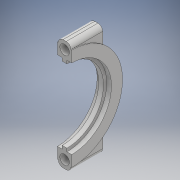
# Autodesk Inventor part: Upper lower eccentric trap (2)
Saved by Autodesk Inventor 2017 (Build 210142000, 142)
## iProperties
Created: 2018-11-20
Part Number: Upper lower eccentric trap (2)
Material: Generic
Document SubType Name: Modeling
Designer: Arman Grewal
Density: 1 g/cm^3
Appearance: Default
Author: Arman Grewal
Autodesk Inventor part; units mm, degrees
ref_plane "XZ Plane" through (0, 0, 0) normal (0, 1, 0) x (-1, 0, 0)
ref_plane "XY Plane" through (0, 0, 0) normal (0, 0, 1) x (1, 0, 0)
sketch "Sketch1" plane through (0, 0, 0) normal (1, 0, 0) x (0, 1, 0)
  arc A0 (0, -16) -> (0, 16) centre (0, 0) ccw construction
  arc A1 (0, -16) -> (0, 16) centre (0, 0) ccw
  arc A2 (0, -12.5) -> (0, 12.5) centre (0, 0) ccw
  line L0 (0, 12.5) -> (0, 16)
  line L1 (0, -12.5) -> (0, -16)
  dimension "d0" = 32
  dimension "d1" = 25
  dimension "d2" = 0
  dimension "d3" = 0
  dimension "d4" = 0
  dimension "d5" = 16
  constraints: 6 point on circle, 4 end point, 3 centre point, 3 coincident, 1 collinear, 1 concentric, 1 vertical
  measures "d0" diameter of A0
  measures "d1" diameter of A2
  measures "d2" distance between parallel lines of L0 L1
  measures "d3" distance from line of point (0, 0) L0
  measures "d4" distance from line of point (0, 0) L0
  measures "d5" distance of point (0, 0) L0.end
extrude "Extrusion1" add sketch "Sketch1" along normal blind 4.5
ref_plane "Work Plane1" through (2.25, 0, 0) normal (1, 0, 0) x (0, 1, 0)
sketch "Sketch3" plane through (2.25, 0, 0) normal (1, 0, 0) x (0, 1, 0)
  arc A0 (0, -12.5) -> (0, 12.5) centre (0, 0) ccw projected
  arc A1 (0, -11.5) -> (0, 11.5) centre (0, 0) ccw
  line L0 (0, -11.5) -> (0, -12.5)
  line L1 (0, 12.5) -> (0, 11.5)
  dimension "d8" = 23
  constraints: 4 end point, 2 point on circle, 2 vertical, 1 centre point, 1 concentric
  measures "d8" diameter of A1
extrude "Extrusion2" add sketch "Sketch3" along normal mid plane 1.5
sketch "Sketch4" plane through (0, 0, 12.5) normal (0, -1, 0) x (1, 0, 0)
  line L0 (3, 0) -> (4.5, 0) construction
  line L1 (4.5, 0) -> (4.5, 2.5) construction
  line L2 (4.5, 3.5) -> (4.5, 0) construction
  line L3 (0, 3.5) -> (4.5, 3.5) construction
  line L4 (2.25, 3.5) -> (2.25, 0) construction
  circle A0 centre (2.25, 2.5) radius 1.5 construction
  circle A1 centre (2.25, 2.5) radius 1.5
  line L5 (2.25, 0) -> (0.25, 0)
  line L6 (0, 0) -> (1.5, 0) projected
  line L7 (0.25, 0) -> (4.25, 0)
  line L8 (2.25, 0) -> (2.25, 5) construction
  line L9 (0.25, 0) -> (0.25, 3.5)
  line L10 (0.25, 0) -> (0.25, 3.5) construction
  line L11 (2.25, 5) -> (1.75, 5)
  line L12 (1.75, 5) -> (2.75, 5)
  arc A2 (1.75, 5) -> (0.25, 3.5) centre (1.75, 3.5) ccw
  line L13 (4.25, 0) -> (4.25, 3.5)
  arc A3 (4.25, 3.5) -> (2.75, 5) centre (2.75, 3.5) ccw
  point P0 (0, -12.5)
  dimension "d11" = 2.5
  dimension "d12" = 3
  dimension "d13" = 2.5
  dimension "d14" = 0
  dimension "d15" = 2
  dimension "d16" = 4
  dimension "d17" = 5
  dimension "d18" = 0.5
  dimension "d19" = 1
  dimension "d20" = 1.5
  dimension "d21" = 1.5
  constraints: 20 end point, 7 point on line, 4 centre point, 4 point on circle, 3 perpendicular, 2 vertical, 1 coincident, 1 concentric, 1 horizontal, 1 midpoint
  measures "d11" distance of L0.end L1.end
  measures "d12" diameter of A0
  measures "d13" distance from line of A0.centre L0
  measures "d14" distance from line of L4.end L0
  measures "d15" distance of L4.end L5.end
  measures "d16" distance of L5.end L7.end
  measures "d17" distance of L4.end L8.end
  measures "d18" distance of L8.end L11.end
  measures "d19" distance of L11.end L12.end
  measures "d20" radius of A2
  measures "d21" radius of A3
extrude "Extrusion3" add sketch "Sketch4" against normal blind 10
extrude "Extrusion5" cut sketch "Sketch4" against normal blind 1000 contours A1
mirror "Mirror2" about plane through (0, 0, 0) normal (0, 0, 1) of "Extrusion3", "Extrusion5"
body "Solid1"
